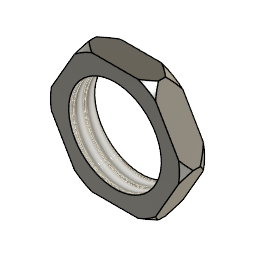
Lock Nut (Autodesk Fusion 360 design; units mm, degrees)
Autodesk Fusion 360 part; units mm, degrees
sketch "Sketch1" plane through (0, 0, 0) normal (0, 1, 0) x (1, 0, 0)
  line L0 (25.4, 0) -> (12.7, 21.997)
  line L1 (12.7, 21.997) -> (-12.7, 21.997)
  line L2 (-12.7, 21.997) -> (-25.4, 0)
  line L3 (-25.4, 0) -> (-12.7, -21.997)
  line L4 (-12.7, -21.997) -> (12.7, -21.997)
  line L5 (12.7, -21.997) -> (25.4, 0)
  dimension "d4" = 25.4
  measures "d4" distance of L0.start origin
extrude "Extrude2" add sketch "Sketch1" along normal blind 9.525
hole "Hole1" at (0, 0, 0) direction (0, 1, 0) diameter 38.1 depth 19.05 tip angle 118
sketch "Sketch3" plane through (0, 0, 0) normal (0, 0, 1) x (1, 0, 0)
  line L0 (-23.2306, 9.525) -> (-25.4, 5.7675)
  line L1 (-25.4, 9.525) -> (-12.7, 9.525)
  line L2 (-25.4, 0) -> (-25.4, 9.525)
  line L3 (-23.5593, 0) -> (-25.4, 3.1882)
  line L4 (-25.4, 0) -> (-12.7, 0)
  dimension "d12" = 150
  dimension "d13" = 150
  constraint coincident L0.start L1
  constraint coincident L0.end L2
  constraint coincident L2 L3.end
  constraint coincident L3.start L4
  measures "d12" angle of L0 L2
  measures "d13" angle of L2 L3
revolve "Revolve1" cut sketch "Sketch3" angle 360 about axis through (0, 0, 0) along (0, 1, 0)
thread "Thread1" "ANSI Unified Screw Threads 1.5 1 1/2-6 UNC 1 1/2-6 UNC 3B" major diameter 38.1 minor diameter 33.7769 pitch 4.2333 angle 60 resizes the face on face at (1.8968, 3.175, -18.9553)
equation "d5 = 3 / 8 * 1 in"
